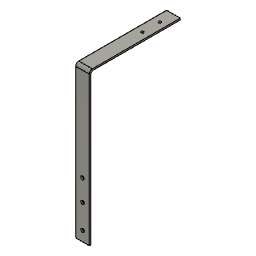
Cable bracket (Autodesk Fusion 360 design; units mm, degrees)
Autodesk Fusion 360 part; units mm, degrees
sketch "Bracket" plane through (0, 0, 0) normal (1, 0, 0) x (0, 1, 0)
  line L0 (0, 0) -> (2, 0)
  line L1 (2, -2) -> (2, -200)
  line L2 (2, -200) -> (0, -200)
  line L3 (0, -200) -> (0, 0)
  line L4 (0, 0) -> (120, 0)
  line L5 (120, 0) -> (120, -2)
  line L6 (120, -2) -> (2, -2)
  line L7 (0, -2) -> (0, 0)
  dimension "d1" = 2
  dimension "d2" = 200
  dimension "d3" = 120
  dimension "d4" = 2
  constraint horizontal L0
  constraint vertical L1
  constraint horizontal L2
  constraint vertical L3
  constraint coincident L0.start L3.end
  constraint horizontal L4
  constraint vertical L5
  constraint horizontal L6
  constraint vertical L7
  measures "d1" distance of L0.start L0.end
  measures "d2" distance of L0.start L2.end
  measures "d3" distance of L0.start L4.end
  measures "d4" distance of L0.start L7.start
extrude "Extrude1" add sketch "Bracket" along normal blind 18
fillet "Fillet1" radius 3 1 edges at (9, 2, -2)
fillet "Fillet2" radius 4 1 edges at (9, 0, 0)
sketch "Front Holes" plane through (0, 0, 0) normal (0, -1, 0) x (1, 0, 0)
  line L0 (18, -4) -> (0, -4)
  line L1 (0, -4) -> (0, -200)
  line L2 (0, -200) -> (18, -200)
  line L3 (18, -200) -> (18, -4)
  line L4 (9, -200) -> (9, -113.9355) construction
  circle A0 centre (9, -187) radius 2.25
  circle A1 centre (9, -155) radius 2.25
  circle A2 centre (9, -127) radius 2.25
  dimension "d9" = 4.5
  dimension "d10" = 4.5
  dimension "d11" = 4.5
  dimension "d12" = 13
  dimension "d13" = 32
  dimension "d14" = 28
  constraint midpoint L2 L4.start
  constraint perpendicular L2 L4
  constraint coincident L4 A0.centre
  constraint coincident L4 A1.centre
  constraint coincident L4 A2.centre
  measures "d9" diameter of A0
  measures "d10" diameter of A1
  measures "d11" diameter of A2
  measures "d12" distance of L2 A0.centre
  measures "d13" distance of A0.centre A1.centre
  measures "d14" distance of A1.centre A2.centre
sketch "Top Holes" plane through (0, 0, 0) normal (0, 0, 1) x (-1, 0, 0)
  line L0 (0, -4) -> (-18, -4)
  line L1 (-18, -4) -> (-18, -120)
  line L2 (-18, -120) -> (0, -120)
  line L3 (0, -120) -> (0, -4)
  line L4 (-9, -120) -> (-9, -16.6564) construction
  circle A0 centre (-9, -102) radius 1.75
  circle A1 centre (-9, -79) radius 1.75
  dimension "d15" = 3.5
  dimension "d16" = 3.5
  dimension "d17" = 18
  dimension "d18" = 23
  constraint midpoint L2 L4.start
  constraint perpendicular L2 L4
  constraint coincident L4 A0.centre
  constraint coincident L4 A1.centre
  measures "d15" diameter of A0
  measures "d16" diameter of A1
  measures "d17" distance of L2 A0.centre
  measures "d18" distance of A0.centre A1.centre
extrude "Extrude2" cut sketch "Front Holes" against normal blind 5 contours A0 | A1 | A2
extrude "Extrude3" cut sketch "Top Holes" against normal blind 5 contours A0 | A1
equation "d10 = d9"
equation "d11 = d9"
equation "d16 = d15"
named bodies: "Bracket"
